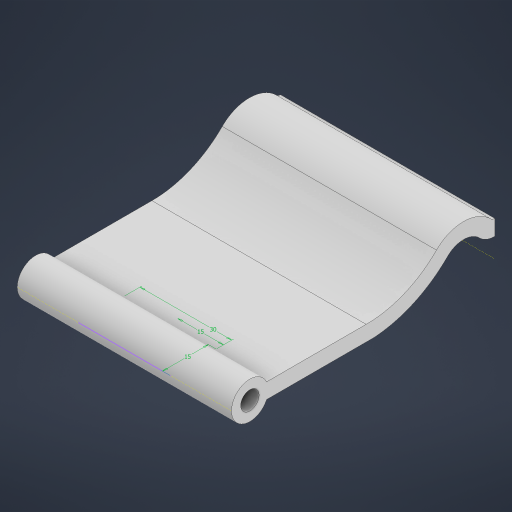
# Autodesk Inventor part: Part2
Saved by Autodesk Inventor 2023 (Build 270158000, 158)
## iProperties
Created: 2022-11-21
Part Number: Part2
Material: Generic
Document SubType Name: Modeling
Designer: iusti
Density: 1 g/cm^3
Appearance: Default
Author: iusti
Autodesk Inventor part; units mm, degrees
ref_plane "YZ Plane" through (0, 0, 0) normal (1, 0, 0) x (0, 1, 0)
ref_plane "XZ Plane" through (0, 0, 0) normal (0, 1, 0) x (-1, 0, 0)
ref_plane "XY Plane" through (0, 0, 0) normal (0, 0, 1) x (1, 0, 0)
sketch "Sketch5" plane through (0, 0, 0) normal (1, 0, 0) x (0, 1, 0)
  line L0 (0, 0) -> (0, -38) construction
  line L1 (0, -38) -> (35, -38) construction
  line L2 (35, -38) -> (3.1802, -69.8198) construction
  arc A0 (0, -38) -> (10.2513, -62.7487) centre (35, -38) ccw construction
  arc A1 (10.2513, -76.8909) -> (10.2513, -62.7487) centre (3.1802, -69.8198) ccw construction
  line L3 (3.1802, -69.8198) -> (13.2918, -79.9314) construction
  arc A2 (10.2513, -76.8909) -> (8.9924, -80) centre (13.2918, -79.9314) ccw construction
  line L4 (2.5, -5.4544) -> (2.5, -38)
  arc A3 (2.5, -38) -> (12.019, -60.981) centre (35, -38) ccw
  arc A4 (12.019, -78.6586) -> (12.019, -60.981) centre (3.1802, -69.8198) ccw
  arc A5 (12.019, -78.6586) -> (11.4931, -80) centre (13.2918, -79.9314) ccw
  line L5 (-2.5, -5.4544) -> (-2.5, -40.4493)
  arc A6 (-2.5, -40.4493) -> (8.427, -64.573) centre (35, -38) ccw
  arc A7 (8.427, -75.0666) -> (8.427, -64.573) centre (3.1802, -69.8198) ccw
  arc A8 (8.427, -75.0666) -> (6.4123, -80) centre (13.2918, -79.9314) ccw
  line L6 (11.4931, -80) -> (6.4123, -80)
  arc A9 (2.5, -5.4544) -> (-2.5, -5.4544) centre (0, 0) ccw
  circle A10 centre (0, 0) radius 3
  dimension "d30" = 35
  dimension "d31" = 45
  dimension "d32" = 45
  dimension "d33" = 14.3
  dimension "d34" = 2.5
  dimension "d35" = 2.5
  dimension "d39" = 12
  dimension "d40" = 6
  dimension "d41" = 38
  dimension "d42" = 80
  constraints: 20 point on circle, 14 end point, 11 centre point, 5 coincident, 4 point on line, 2 perpendicular, 1 horizontal, 1 vertical, 4 other
  measures "d30" distance of L0.end L1.end
  measures "d31" angle of L1 L2
  measures "d32" distance of L2.end A0.centre
  measures "d33" distance of L3.start L3.end
  measures "d34" distance between parallel lines of L0 L4
  measures "d35" distance between parallel lines of L0 L5
  measures "d39" diameter of A9
  measures "d40" diameter of A10
  measures "d41" distance of L0.end L0.start
  measures "d42" vertical distance of L6.end L0.start
extrude "Extrusion2" add sketch "Sketch5" along normal mid plane 70
sketch "Sketch6" plane through (0, 0, 0) normal (0, 1, 0) x (-1, 0, 0)
  line L0 (35, -80) -> (-35, -80) construction
  line L1 (0, -80) -> (0, 6) construction
  line L2 (35, 6) -> (-35, 6) construction
  line L3 (15, -9) -> (-15, -9)
  line L4 (-15, -9) -> (-15, 6)
  line L5 (-15, 6) -> (15, 6)
  line L6 (15, 6) -> (15, -9)
  point P0 (0, 0)
  dimension "d43" = 30
  dimension "d44" = 15
  dimension "d45" = 15
  constraints: 10 end point, 2 midpoint, 2 parallel, 1 horizontal, 1 perpendicular
  measures "d43" distance of L3.start L3.end
  measures "d44" distance from line of L3.end L1
  measures "d45" distance of L3.end L4.end
body "Solid3"
